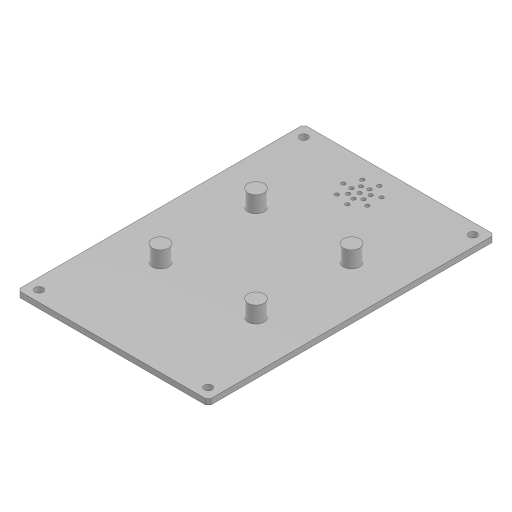
# Autodesk Inventor part: Case_bottom
Saved by Autodesk Inventor 2023.1 (Build 271208000, 208)
## iProperties
Created: 2022-08-03
Part Number: Case_bottom
Material: PC/ABS-Kunststoff
Document SubType Name: Modeling
Designer: tland
Density: 0.357273 g/cm^3
Appearance: Glatt - Mittelgrau
Author: tland
Autodesk Inventor part; units mm, degrees
ref_plane "YZ Plane" through (0, 0, 0) normal (1, 0, 0) x (0, 1, 0)
ref_plane "XZ Plane" through (0, 0, 0) normal (0, 1, 0) x (-1, 0, 0)
ref_plane "XY Plane" through (0, 0, 0) normal (0, 0, 1) x (1, 0, 0)
sketch "Skizze1" plane through (0, 0, 0) normal (0, 1, 0) x (-1, 0, 0)
  line L0 (35, 52.5) -> (-35, 52.5)
  line L1 (-35, 52.5) -> (-35, -52.5)
  line L2 (-35, -52.5) -> (35, -52.5)
  line L3 (35, -52.5) -> (35, 52.5)
  point P0 (0, 0)
  point P1 (35, 0)
  point P2 (0, 52.5)
  dimension "d0" = 70
  dimension "d1" = 105
  constraints: 8 end point, 2 midpoint, 2 parallel, 1 horizontal, 1 horizontal alignment, 1 perpendicular, 1 vertical alignment
  measures "d0" distance of L0.start L0.end
  measures "d1" distance of L2.end L0.start
extrude "Extrusion1" add sketch "Skizze1" along normal blind 2
sketch "Skizze3" plane through (0, 2, 0) normal (0, 1, 0) x (1, 0, 0)
  line L0 (31, 48.5) -> (-31, 48.5) construction
  line L1 (-31, 48.5) -> (-31, -48.5) construction
  line L2 (-31, -48.5) -> (31, -48.5) construction
  line L3 (31, -48.5) -> (31, 48.5) construction
  line L4 (35, -52.5) -> (35, 52.5) construction
  line L5 (35, 52.5) -> (-35, 52.5) construction
  line L6 (-35, 52.5) -> (-35, -52.5) construction
  line L7 (-35, -52.5) -> (35, -52.5) construction
  point P0 (0, 0)
  point P1 (31, 0)
  point P2 (0, 48.5)
  dimension "d27" = 105
  dimension "d28" = 70
  dimension "d29" = 62
  dimension "d30" = 97
  constraints: 8 end point, 4 coincident, 2 midpoint, 2 parallel, 1 horizontal, 1 horizontal alignment, 1 perpendicular, 1 vertical alignment
  measures "d27" distance of L5.end L6.end
  measures "d28" distance of L6.end L4.start
  measures "d29" distance of L1.end L2.end
  measures "d30" distance of L0.end L1.end
hole "Bohrung1" at (31, 2, 48.5) at (-31, 2, 48.5) at (-31, 2, -48.5) at (31, 2, -48.5) direction (0, -1, 0) diameter 3 end through all
sketch "Skizze5" plane through (0, 2, 0) normal (0, 1, 0) x (1, 0, 0)
  line L0 (0, 40.5) -> (-2, 40.5)
  line L1 (-2, 40.5) -> (-2, 20.5)
  line L2 (-2, 20.5) -> (0, 20.5)
  line L3 (0, 20.5) -> (0, 40.5)
  line L4 (0, 10.5) -> (-7, 10.5)
  line L5 (-7, 10.5) -> (-7, 8.5)
  line L6 (-7, 8.5) -> (0, 8.5)
  line L7 (0, 8.5) -> (0, 10.5)
  circle A0 centre (-31, 48.5) radius 1.5 construction
  circle A1 centre (31, -48.5) radius 1.5 construction
  circle A2 centre (-31, -48.5) radius 1.5 construction
  circle A3 centre (31, 48.5) radius 1.5 construction
  line L8 (35, -52.5) -> (35, 52.5) construction
  line L9 (35, 52.5) -> (-35, 52.5) construction
  line L10 (-35, 52.5) -> (-35, -52.5) construction
  line L11 (-35, -52.5) -> (35, -52.5) construction
  line L12 (-7, 20.5) -> (-5, 20.5)
  line L13 (-5, 20.5) -> (-5, 40.5)
  line L14 (-5, 40.5) -> (-7, 40.5)
  line L15 (-7, 40.5) -> (-7, 20.5)
  point P0 (0, 0)
  point P1 (-1, 20.5)
  dimension "d45" = 2
  dimension "d46" = 42
  dimension "d48" = 20
  dimension "d49" = 7
  dimension "d51" = 0
  dimension "d56" = 10
  dimension "d57" = 3
  dimension "d58" = 20
  dimension "d59" = 0
  constraints: 24 end point, 6 parallel, 3 horizontal, 3 perpendicular, 2 equal length, 1 midpoint, 1 point on line
  measures "d45" distance of L0.start L0.end
  measures "d46" distance between parallel lines of L9 L4
  measures "d48" distance of L2.end L0.start
  measures "d49" distance of L5.end L6.end
  measures "d51" distance from line of L3 point (0, 0)
  measures "d56" distance between parallel lines of L4 L2
  measures "d57" distance between parallel lines of L1 L13
  measures "d58" distance of L14.end L12.start
  measures "d59" distance between parallel lines of L2 L12
extrude "Extrusion5" [suppressed]
sketch "Skizze6" plane through (0, 2, 0) normal (0, 1, 0) x (1, 0, 0)
  line L0 (-17.5, 17.5) -> (17.5, 17.5) construction
  line L1 (17.5, 17.5) -> (17.5, -17.5) construction
  line L2 (17.5, -17.5) -> (-17.5, -17.5) construction
  line L3 (-17.5, -17.5) -> (-17.5, 17.5) construction
  circle A0 centre (-17.5, 17.5) radius 3
  circle A1 centre (-17.5, -17.5) radius 3
  circle A2 centre (17.5, -17.5) radius 3
  circle A3 centre (17.5, 17.5) radius 3
  point P0 (0, 0)
  point P1 (-17.5, 0)
  point P2 (0, 17.5)
  dimension "d60" = 35
  dimension "d61" = 6
  dimension "d62" = 6
  dimension "d63" = 6
  dimension "d64" = 6
  constraints: 8 end point, 4 centre point, 4 coincident, 2 midpoint, 2 parallel, 2 perpendicular, 1 horizontal, 1 horizontal alignment, 1 vertical alignment
  measures "d60" distance of L2.end L0.start
  measures "d61" diameter of A0
  measures "d62" diameter of A1
  measures "d63" diameter of A2
  measures "d64" diameter of A3
extrude "Extrusion6" add sketch "Skizze6" along normal blind 6
sketch "Skizze7" plane through (0, 0, 0) normal (0, -1, 0) x (1, 0, 0)
  circle A0 centre (-17.5, 17.5) radius 3 construction
  circle A1 centre (-17.5, -17.5) radius 3 construction
  arc A2 (20.5, -17.5) -> (20.5, -17.5) centre (17.5, -17.5) ccw construction
  arc A3 (20.5, 17.5) -> (20.5, 17.5) centre (17.5, 17.5) ccw construction
  point P0 (0, 0)
  point P1 (20, -17.5)
  point P2 (20, 17.5)
  constraints: 4 coincident, 2 other
hole "Bohrung2" at (-17.5, 0, 17.5) at (-17.5, 0, -17.5) at (17.5, 0, -17.5) at (17.5, 0, 17.5) direction (0, 1, 0) diameter 2.5 depth 5 tip angle 118
chamfer "Fase1" distance 1 angle 45 4 edges at (-35, 1, 52.5) (35, 1, 52.5) (35, 1, -52.5) (-35, 1, -52.5)
sketch "Skizze10" plane through (0, 0, 0) normal (0, -1, 0) x (1, 0, 0)
  point P0 (0, 0)
  point P1 (-3, -41)
  point P2 (-6, -41)
  point P3 (-9, -41)
  dimension "d105" = 41
  dimension "d106" = 3
  dimension "d107" = 3
  dimension "d108" = 3
  constraints: 2 horizontal alignment
  measures "d105" vertical distance of point (0, 0) point (-3, -41)
  measures "d106" horizontal distance of point (0, 0) point (-3, -41)
  measures "d107" distance of point (-3, -41) point (-6, -41)
  measures "d108" distance of point (-9, -41) point (-6, -41)
hole "Bohrung3" at (-3, 0, -41) at (-6, 0, -41) at (-9, 0, -41) direction (0, 1, 0) diameter 1.5 depth 5 tip angle 118
pattern_circular "Runde Anordnung1" count 7 over 360 about axis through (-3, 2.5, -41) along (0, -1, 0) of "Bohrung3"
equation "\"d62\" = d61"
equation "\"d63\" = d61"
equation "\"d64\" = d61"
